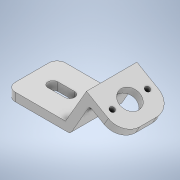
# Autodesk Inventor part: 1번
Saved by Autodesk Inventor 2022 (Build 260153000, 153)
## iProperties
Created: 2021-09-04
Part Number: 1번
Material: 일반
Document SubType Name: Modeling
Designer: 서울공업고등학교
Density: 1 g/cm^3
Appearance: 기본값
Author: 서울공업고등학교
Autodesk Inventor part; units mm, degrees
ref_plane "YZ Plane" through (0, 0, 0) normal (1, 0, 0) x (0, 1, 0)
ref_plane "XZ Plane" through (0, 0, 0) normal (0, 1, 0) x (-1, 0, 0)
ref_plane "XY Plane" through (0, 0, 0) normal (0, 0, 1) x (1, 0, 0)
sketch "스케치1" plane through (0, 0, 0) normal (0, 0, 1) x (1, 0, 0)
  line L0 (0, 0) -> (0, -10)
  line L1 (0, -10) -> (75.7735, -10)
  line L2 (0, 0) -> (70, 0)
  line L3 (0, 0) -> (70, 0) construction
  line L4 (70, 0) -> (95, 43.3013)
  line L5 (95, 43.3013) -> (138.3013, 18.3013)
  line L6 (138.3013, 18.3013) -> (133.3013, 9.641)
  line L7 (133.3013, 9.641) -> (98.6603, 29.641)
  line L8 (98.6603, 29.641) -> (75.7735, -10)
  dimension "d0" = 10
  dimension "d10" = 70
  dimension "d12" = 50
  dimension "d13" = 120
  dimension "d14" = 50
  dimension "d15" = 90
  dimension "d16" = 10
  dimension "d17" = 90
  dimension "d18" = 10
  constraints: 18 end point, 4 perpendicular, 2 horizontal, 1 collinear, 1 parallel, 1 vertical
  measures "d0" distance of L0.start L0.end
  measures "d10" distance of L0.start L2.end
  measures "d12" distance of L2.end L4.end
  measures "d13" angle of L4 L2
  measures "d14" distance of L4.end L5.end
  measures "d15" angle of L4 L5
  measures "d16" distance of L5.end L6.end
  measures "d17" angle of L5 L6
  measures "d18" distance between parallel lines of L8 L4
extrude "돌출1" add sketch "스케치1" along normal mid plane 60
fillet "모깎기1" radius 10 2 edges at (0, -5, 30) (0, -5, -30)
fillet "모깎기2" radius 20 2 edges at (135.8013, 13.9711, 30) (135.8013, 13.9711, -30)
fillet "모깎기3" radius 5 1 edges at (75.7735, -10, 0)
fillet "모깎기4" radius 3 1 edges at (98.6603, 29.641, 0)
sketch "스케치2" plane through (70, 0, 30) normal (0, 1, 0) x (1, 0, 0)
  line L0 (-45, 30) -> (-25, 30) construction
  line L1 (-45, 24) -> (-25, 24)
  line L2 (-25, 36) -> (-45, 36)
  arc A0 (-45, 36) -> (-45, 24) centre (-45, 30) ccw
  arc A1 (-25, 24) -> (-25, 36) centre (-25, 30) ccw
  line L3 (-70, 10) -> (-70, 50) projected
  line L4 (0, 0) -> (-60, 0) projected
  point P0 (-70, 30)
  point P1 (-35, 30)
  dimension "d23" = 12
  dimension "d24" = 20
  dimension "d25" = 25
  dimension "d26" = 30
  constraints: 8 end point, 4 point on circle, 4 tangent, 2 centre point, 1 horizontal, 1 midpoint, 1 parallel
  measures "d23" diameter of A1
  measures "d24" distance of L2.start L2.end
  measures "d25" distance from line of L0.start L3
  measures "d26" distance from line of point (-35, 30) L4
extrude "돌출2" cut sketch "스케치2" against normal blind 60
sketch "스케치3" plane through (95, 43.3013, 30) normal (0.5, 0.866, 0) x (0.866, -0.5, 0)
  circle A0 centre (25, 30) radius 12
  circle A1 centre (25, 51) radius 3
  circle A2 centre (25, 9) radius 3
  line L0 (0, 60) -> (0, 0) projected
  line L1 (0, 60) -> (30, 60) projected
  point P0 (-60.6218, 30)
  dimension "d29" = 24
  dimension "d30" = 6
  dimension "d32" = 6
  dimension "d33" = 21
  dimension "d34" = 21
  dimension "d36" = 25
  dimension "d37" = 25
  dimension "d38" = 30
  constraints: 3 centre point
  measures "d29" diameter of A0
  measures "d30" diameter of A1
  measures "d32" diameter of A2
  measures "d33" distance of A0.centre A1.centre
  measures "d34" distance of A0.centre A2.centre
  measures "d36" distance from line of L0 A0.centre
  measures "d37" distance from line of L0 A1.centre
  measures "d38" distance from line of A0.centre L1
extrude "돌출3" cut sketch "스케치3" against normal blind 60
